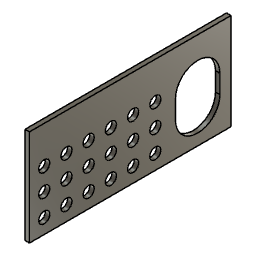
plate_1 v2 (Autodesk Fusion 360 design; units mm, degrees)
Autodesk Fusion 360 part; units mm, degrees
sketch "Sketch1" plane through (0, 0, 0) normal (1, 0, 0) x (0, 1, 0)
  line L0 (0, 0) -> (272.2, 0)
  line L1 (272.2, 0) -> (272.2, 130)
  line L2 (272.2, 130) -> (0, 130)
  line L3 (0, 130) -> (0, 0)
  dimension "d1" = 272.2
  dimension "d2" = 130
  constraint horizontal L0
  constraint vertical L1
  constraint horizontal L2
  constraint vertical L3
  constraint coincident L0.start L3.end
  measures "d1" distance of L0.start L0.end
  measures "d2" distance of L0.start L2.end
extrude "Extrude1" add sketch "Sketch1" against normal blind 6
sketch "Sketch2" plane through (0, 0, 0) normal (1, 0, 0) x (0, 1, 0)
  line L0 (0, 130) -> (0, 0)
  line L1 (0, 0) -> (272.2, 0)
  line L2 (272.2, 0) -> (272.2, 130)
  line L3 (272.2, 130) -> (0, 130)
  line L4 (257.2, 45) -> (257.2, 70)
  arc A0 (257.2, 70) -> (197.2, 70) centre (227.2, 70) ccw
  line L5 (197.2, 70) -> (197.2, 45)
  arc A1 (197.2, 45) -> (257.2, 45) centre (227.2, 45) ccw
  line L6 (227.2, 15) -> (227.2, 100) construction
  circle A2 centre (20, 80) radius 7.5
  circle A3 centre (50, 80) radius 7.5
  circle A4 centre (80, 80) radius 7.5
  circle A5 centre (110, 80) radius 7.5
  circle A6 centre (140, 80) radius 7.5
  circle A7 centre (170, 80) radius 7.5
  circle A8 centre (20, 50) radius 7.5
  circle A9 centre (50, 50) radius 7.5
  circle A10 centre (80, 50) radius 7.5
  circle A11 centre (110, 50) radius 7.5
  circle A12 centre (140, 50) radius 7.5
  circle A13 centre (170, 50) radius 7.5
  circle A14 centre (20, 20) radius 7.5
  circle A15 centre (50, 20) radius 7.5
  circle A16 centre (80, 20) radius 7.5
  circle A17 centre (110, 20) radius 7.5
  circle A18 centre (140, 20) radius 7.5
  circle A19 centre (170, 20) radius 7.5
  dimension "d5" = 60
  dimension "d6" = 15
  dimension "d7" = 15
  constraint tangent L4 A0
  constraint tangent A0 L5
  constraint parallel L4 L5
  constraint tangent L5 A1
  constraint tangent L4 A1
  constraint midpoint A1 L6.start
  constraint midpoint A0 L6.end
  constraint perpendicular L3 L6
  measures "d5" diameter of A0
  measures "d6" distance of L1 L6.start
  measures "d7" distance of L2 L4
extrude "Extrude2" cut sketch "Sketch2" against normal up to surface (6 mm away) contours L4 A0 L5 A1 | A2 | A3 | A4 | A5 | A6 | A7 | A8 | A9 | A10 | A11 | A12 | A13 | A14 | A15 | A16 | A17 | A18 | A19
